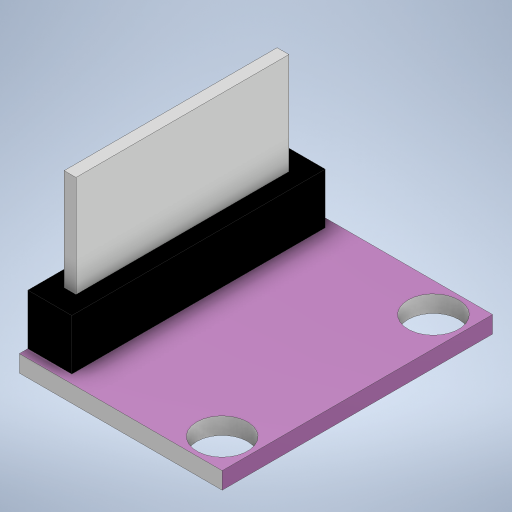
# Autodesk Inventor part: SensorPresionHumedadTemp
Saved by Autodesk Inventor 2024 (Build 280153000, 153)
## iProperties
Created: 2024-05-18
Part Number: SensorPresionHumedadTemp
Material: Genérico
Document SubType Name: Modeling
Designer: alexa
Density: 1 g/cm^3
Appearance: Valor por defecto
Author: alexa
Autodesk Inventor part; units mm, degrees
ref_plane "YZ Plane" through (0, 0, 0) normal (1, 0, 0) x (0, 1, 0)
ref_plane "XZ Plane" through (0, 0, 0) normal (0, 1, 0) x (-1, 0, 0)
ref_plane "XY Plane" through (0, 0, 0) normal (0, 0, 1) x (1, 0, 0)
sketch "Sketch1" plane through (0, 0, 0) normal (0, 1, 0) x (-1, 0, 0)
  line L0 (-6, 8) -> (6, 8)
  line L1 (6, 8) -> (6, -8)
  line L2 (6, -8) -> (-6, -8)
  line L3 (-6, -8) -> (-6, 8)
  line L4 (-6, 8) -> (6, -8) construction
  line L5 (6, 8) -> (-6, -8) construction
  line L6 (-6, 8) -> (-4.25, 8)
  line L7 (-6, 6.25) -> (-6, 8)
  circle A0 centre (-4.25, 6.25) radius 1.5
  line L8 (0, 0) -> (-1.7804, 0)
  circle A1 centre (-4.25, -6.25) radius 1.5
  dimension "d0" = 12
  dimension "d1" = 16
  dimension "d4" = 3
  dimension "d7" = 1.75
  constraints: 18 end point, 3 horizontal, 2 centre point, 2 midpoint, 2 parallel, 1 perpendicular, 1 symmetric about line, 1 other
  measures "d0" distance of L1.end L2.end
  measures "d1" distance of L0.end L1.end
  measures "d4" diameter of A0
  measures "d7" horizontal distance of L2.end A1.centre
extrude "Extrusion1" add sketch "Sketch1" along normal blind 1
sketch "Sketch2" plane through (0, 1, 0) normal (0, 1, 0) x (1, 0, 0)
  line L0 (-6, 8) -> (-6, -8) projected
  line L1 (-3.4, 7.5) -> (-6, 7.5)
  line L2 (-6, 7.5) -> (-6, -7.5)
  line L3 (-6, -7.5) -> (-3.4, -7.5)
  line L4 (-3.4, -7.5) -> (-3.4, 7.5)
  line L5 (-3.4, 7.5) -> (-6, -7.5) construction
  line L6 (-6, 7.5) -> (-3.4, -7.5) construction
  point P0 (0, 0)
  dimension "d9" = 2.6
  dimension "d10" = 15
  constraints: 12 end point, 2 parallel, 1 horizontal, 1 perpendicular
  measures "d9" distance of L3.end L2.end
  measures "d10" distance of L2.end L1.end
extrude "Extrusion2" add sketch "Sketch2" along normal blind 3
sketch "Sketch3" plane through (0, 4, 0) normal (0, 1, 0) x (1, 0, 0)
  line L0 (-6, -7.5) -> (-6, -8) projected
  line L1 (-6, 7.5) -> (-3.4, 7.5) projected
  line L2 (-6, 7.5) -> (-6, -7.5) projected
  line L3 (-3.4, -7.5) -> (-3.4, 7.5) projected
  line L4 (-4.35, -6.3) -> (-5.05, -6.3)
  line L5 (-5.05, -6.3) -> (-5.05, 6.3)
  line L6 (-5.05, 6.3) -> (-4.35, 6.3)
  line L7 (-4.35, 6.3) -> (-4.35, -6.3)
  line L8 (-4.35, -6.3) -> (-5.05, 6.3) construction
  line L9 (-5.05, -6.3) -> (-4.35, 6.3) construction
  point P0 (0, 0)
  point P1 (-4.7, 0)
  dimension "d13" = 12.6
  dimension "d14" = 0.7
  constraints: 12 end point, 2 midpoint, 2 parallel, 1 horizontal, 1 perpendicular
  measures "d13" distance of L4.end L5.end
  measures "d14" distance between parallel lines of L7 L5
extrude "Extrusion3" add sketch "Sketch3" along normal blind 6
body "Solid1"
